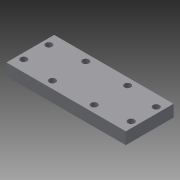
# Autodesk Inventor part: casterplate
Saved by Autodesk Inventor 2015 (Build 190159000, 159)
## iProperties
Created: 2014-12-03
Part Number: casterplate
Material: Generic
Document SubType Name: Modeling
Designer: ericd_000
Density: 1 g/cm^3
Appearance: Default
Author: ericd_000
Autodesk Inventor part; units mm, degrees
ref_plane "YZ Plane" through (0, 0, 0) normal (1, 0, 0) x (0, 1, 0)
ref_plane "XZ Plane" through (0, 0, 0) normal (0, 1, 0) x (-1, 0, 0)
ref_plane "XY Plane" through (0, 0, 0) normal (0, 0, 1) x (1, 0, 0)
sketch "Sketch1" plane through (0, 0, 0) normal (0, 0, 1) x (1, 0, 0)
  line L0 (-50, 20) -> (50, 20)
  line L1 (50, 20) -> (50, -20)
  line L2 (50, -20) -> (-50, -20)
  line L3 (-50, -20) -> (-50, 20)
  circle A0 centre (-45, 10.5) radius 2.75
  circle A1 centre (-45, -10.5) radius 2.75
  circle A2 centre (45, 10.5) radius 2.75
  circle A3 centre (45, -10.5) radius 2.75
  line L4 (-45, 10.5) -> (-45, -10.5) construction
  point P0 (0, 0)
  point P1 (-50, 0)
  point P2 (0, 20)
  point P3 (-45, 0)
  dimension "d0" = 40
  dimension "d1" = 100
  dimension "d2" = 5.5
  dimension "d3" = 5.5
  dimension "d4" = 5
  dimension "d7" = 5
  dimension "d10" = 90
  dimension "d29" = 21
  constraints: 10 end point, 4 centre point, 3 midpoint, 2 horizontal, 2 horizontal alignment, 2 parallel, 1 perpendicular, 1 vertical alignment, 4 other
  measures "d0" distance of L2.end L0.start
  measures "d1" distance of L0.start L0.end
  measures "d2" diameter of A0
  measures "d3" diameter of A1
  measures "d4" distance from line of L3 L4.start
  measures "d7" distance from line of L3 L4.end
  measures "d10" distance of L4.start A2.centre
  measures "d29" distance of L4.start L4.end
sketch "Sketch2" plane through (0, 0, 0) normal (0, 0, 1) x (1, 0, 0)
  circle A0 centre (-17.5, 14) radius 2.75
  circle A1 centre (17.5, 14) radius 2.75
  line L0 (-17.5, 14) -> (17.5, 14) construction
  line L1 (0, 0) -> (0, 14) construction
  circle A2 centre (-17.5, -14) radius 2.75
  circle A3 centre (17.5, -14) radius 2.75
  dimension "d15" = 5.5
  dimension "d17" = 5.5
  dimension "d20" = 35
  dimension "d21" = 14
  dimension "d24" = 28
  constraints: 4 centre point, 4 end point, 2 vertical, 1 horizontal, 1 midpoint, 1 vertical alignment, 4 other
  measures "d15" diameter of A0
  measures "d17" diameter of A1
  measures "d20" distance of L0.start L0.end
  measures "d21" distance of L1.end L1.start
  measures "d24" distance of L0.start A2.centre
extrude "Extrusion1" add sketch "Sketch1" against normal blind 10
extrude "Extrusion2" cut sketch "Sketch2" against normal through all
body "Solid1"
